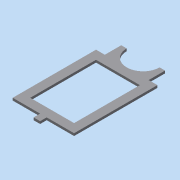
# Autodesk Inventor part: anillo4
Saved by Autodesk Inventor 2015 (Build 190159000, 159)
## iProperties
Created: 2017-09-29
Part Number: anillo4
Material: Generic
Document SubType Name: Modeling
Designer: macbook
Density: 1 g/cm^3
Appearance: Default
Author: macbook
Autodesk Inventor part; units mm, degrees
ref_plane "YZ Plane" through (0, 0, 0) normal (1, 0, 0) x (0, 1, 0)
ref_plane "XZ Plane" through (0, 0, 0) normal (0, 1, 0) x (-1, 0, 0)
ref_plane "XY Plane" through (0, 0, 0) normal (0, 0, 1) x (1, 0, 0)
sketch "Sketch1" plane through (0, 0, 0) normal (0, 0, 1) x (1, 0, 0)
  line L0 (0, 0) -> (100, 0)
  line L1 (100, 0) -> (100, 150)
  line L2 (100, 150) -> (0, 150)
  line L3 (0, 150) -> (0, 0)
  circle A0 centre (50, 207.5) radius 37.5
  line L4 (-20, -20) -> (120, -20)
  line L5 (120, -20) -> (120, 170)
  line L6 (120, 170) -> (-20, 170)
  line L7 (-20, 170) -> (-20, -20)
  line L8 (0, 170) -> (100, 170)
  line L9 (49.5, -20) -> (59.5, -20)
  line L10 (45, -20) -> (60, -20)
  line L11 (42.5, -20) -> (57.5, -20)
  line L12 (57.5, -20) -> (57.5, -35)
  line L13 (57.5, -35) -> (42.5, -35)
  line L14 (42.5, -35) -> (42.5, -20)
  line L15 (100, 170) -> (100, 207.5)
  line L16 (100, 207.5) -> (87.5, 207.5)
  line L17 (0, 170) -> (0, 207.5)
  line L18 (0, 207.5) -> (12.5, 207.5)
  dimension "d0" = 75
  dimension "d1" = 140
  dimension "d3" = 15
  dimension "d4" = 15
  constraints: 38 end point, 6 horizontal, 6 parallel, 5 perpendicular, 4 point on line, 2 point on circle, 2 vertical, 1 centre point
  measures "d0" diameter of A0
  measures "d1" distance of L7.start L5.end
  measures "d3" distance of L12.end L13.end
  measures "d4" distance of L11.end L12.end
extrude "Extrusion1" add sketch "Sketch1" along normal blind 5.5 contours L16 L15 L6 A0 | A0 L6 L17 L18 | L6 L5 L4 L7 | L4 L12 L13 L14
body "Solid1"
